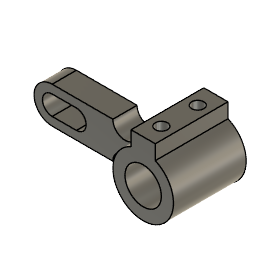
ISO 8 (Autodesk Fusion 360 design; units mm, degrees)
part number: 2025-12-18-11-41-41-177
Autodesk Fusion 360 part; units mm, degrees
sketch "Sketch1" plane through (0, 0, 0) normal (0, 1, 0) x (1, 0, 0)
  arc A0 (-40, 15) -> (-40, -15) centre (-40, 0) ccw
  line L0 (35, -15) -> (35, 15)
  line L1 (-40, -8) -> (-20, -8)
  arc A1 (-20, -8) -> (-20, 8) centre (-20, 0) ccw
  line L2 (-20, 8) -> (-40, 8)
  arc A2 (-40, 8) -> (-40, -8) centre (-40, 0) ccw
  line L3 (-40, 0) -> (-20, 0) construction
  line L4 (-40, -15) -> (10, -15)
  line L5 (30, -15) -> (35, -15)
  arc A3 (30, -15) -> (10, -15) centre (20, -15) ccw
  line L6 (-40, 15) -> (10, 15)
  line L7 (30, 15) -> (35, 15)
  arc A4 (10, 15) -> (30, 15) centre (20, 15) ccw
  dimension "d1" = 30
  dimension "d2" = 75
  dimension "d3" = 75
  dimension "d4" = 20
  dimension "d5" = 16
  dimension "d7" = 20
  dimension "d8" = 20
  constraint horizontal L6
  constraint horizontal L4
  constraint perpendicular L0 L6
  constraint tangent L1 A1
  constraint tangent A1 L2
  constraint parallel L1 L2
  constraint tangent L2 A2
  constraint tangent L1 A2
  constraint horizontal L3
  constraint coincident A0.centre A2.centre
  constraint coincident A4.centre L6
  constraint coincident A3.centre L4
  constraint collinear L4 L5
  constraint collinear L6 L7
  measures "d1" diameter of A0
  measures "d2" distance of A0.start L0.end
  measures "d3" distance of A0.end L0.start
  measures "d4" distance of A0.centre A1.centre
  measures "d5" diameter of A1
  measures "d7" diameter of A4
  measures "d8" diameter of A3
extrude "Extrude1" add sketch "Sketch1" along normal mid plane 20 makes body 1
sketch "Sketch2" plane through (0, 0, 0) normal (0, 1, 0) x (1, 0, 0)
  circle A0 centre (55, 0) radius 15
  line L0 (55, -35) -> (45, -35)
  line L1 (55, -35) -> (65, -35)
  line L2 (45, -35) -> (45, -22.9129)
  line L3 (65, -35) -> (65, -22.9129)
  arc A1 (65, -22.9129) -> (45, -22.9129) centre (55, 0) ccw
  dimension "d13" = 30
  dimension "d14" = 35
  constraint concentric A0 A1
  constraint perpendicular L0 L2
  constraint perpendicular L0 L3
  measures "d13" diameter of A0
  measures "d14" distance of A0.centre L0.start
extrude "Extrude2" add sketch "Sketch2" along normal mid plane 60 separate body makes body 2
sketch "Sketch3" plane through (0, 0, 35) normal (0, 0, 1) x (-1, 0, 0)
  line L0 (-65, 30) -> (-65, -30)
  line L1 (-65, -30) -> (-45, -30)
  line L2 (-45, -30) -> (-45, 30)
  line L3 (-45, 30) -> (-65, 30)
  circle A0 centre (-55, -15) radius 5
  circle A1 centre (-55, 15) radius 5
  dimension "d17" = 10
  dimension "d18" = 10
  measures "d17" diameter of A0
  measures "d18" diameter of A1
extrude "Extrude3" cut sketch "Sketch3" against normal blind 25 contours A0 | A1 bodies 2
